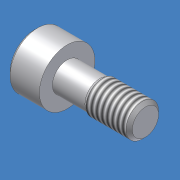
# Autodesk Inventor part: HCBST5-12_Screw
Saved by Autodesk Inventor 2014 SP1 (Build 180222100, 222)
## iProperties
Category: PARTsolutions
Created: 2015-02-04
Part Number: HCBST5-12_Screw
Catalog Web Link: www.cadenas.de
Description: HCBSTscrew - Frame Washer Assembled Hexagon Socket Head Cap Screws for Aluminum Frames
Document SubType Name: Modeling
Designer: PARTsolutions
Material: Generic
Density: 1 g/cm^3
Appearance: RGB(192,192,192)
NB: HCBST5-12_Screw
NN: HCBSTscrew
NT: Frame Washer Assembled Hexagon Socket Head Cap Screws for Aluminum Frames
NBSYN: $PN.
LINA: HCBST5-12_Screw
PN: HCBST5-12_Screw
TYPE: HCBST
MATB: Structural Alloy Steel
HARD: 32~44HRC
MATSW: JIS B1251
MATFW: JIS B1256
ST: Trivalent Chromate
M: 5
L: 12
M1: 5.000
L0: 12,16
NDM: 5.000
KDM: 4.017
MP: 5X0.8
P: 0.800
A: 8.5
E: 5
B: 4
C: 8.5
D: 10.0
AA: 5.4
KT: DUMMY
SUPPLIER: Misumi
ARTICLENO: HCBST5-12_Screw
BOMINFO: HCBST5-12_Screw
CREATOR: CADENAS GmbH
PSOL_IDENT_0: {\\10.0.0.236\data_v8\23d-libs\misumi\metric\38_al_extrusions_blackets\nuts\hcbst_screw.prj},177 {VT
PSOL_IDENT_1: YP=3D},{NB=HCBST5-12_Screw},{LINA=HCBST5-12_Screw},{NN=HCBSTscrew},{DATE=19.11.2014 02:34:01},{GEOMD
PSOL_IDENT_2: ATE=24.08.2009 08:32:00},{VERSION=},{LINEID=40},{LINESUBID=-1},{WBVAR=L}  {NB=HCBST5-12_Screw},{LINA
PSOL_IDENT_3: =HCBST5-12_Screw},{KT=DUMMY},{PN=HCBST5-12_Screw},{TYPE=HCBST},{MATB=Structural Alloy Steel},{HARD=3
PSOL_IDENT_4: 2~44HRC},{MATSW=JIS B1251},{MATFW=JIS B1256},{ST=Trivalent Chromate},{M=5},{L=12},{M1=5.000},{L0=12,
PSOL_IDENT_5: 16},{NDM=5},{KDM=4.017064},{MP=5X0.8},{P=0.8},{A=8.5},{E=5},{B=4},{C=8.5},{D=10.0},{AA=5.4}
Title: HCBST5-12_Screw
Author: Cadenas PARTsolutions
Comments: Frame Washer Assembled Hexagon Socket Head Cap Screws for Aluminum Frames
Autodesk Inventor part; units mm, degrees
sketch "Sketch_6" plane through (0, 0, 0) normal (0, 0, 1) x (1, 0, 0)
  line L0 (12, 0) -> (4.5504, 0)
  line L1 (4.5504, 0) -> (4.5504, 2.0095)
  line L2 (4.5504, 2.0095) -> (5.4, 2.5)
  line L3 (5.4, 2.5) -> (11.5095, 2.5)
  line L4 (11.5095, 2.5) -> (12, 2.0095)
  line L5 (12, 2.0095) -> (12, 0)
  line L6 (12, 0) -> (4.5504, 0)
  constraints: 14 end point
revolve "Revolution1" add sketch "Sketch_6" angle 360 about axis through (12, 0, 0) along (1, 0, 0)
thread "Thread1" size "M5x0.8" class "6g" standard "ISO Metric profile" full length
sketch "Sketch_1" plane through (0, 0, 0) normal (0, 0, 1) x (1, 0, 0)
  line L0 (5.4, 0) -> (-5, 0)
  line L1 (-1.3453, 0) -> (-2.5, 2)
  line L2 (-2.5, 2) -> (-5, 2)
  line L3 (-5, 2) -> (-5, 3.75)
  line L4 (-5, 3.75) -> (-4.5, 4.25)
  line L5 (-4.5, 4.25) -> (0, 4.25)
  line L6 (0, 4.25) -> (0, 2.2543)
  line L7 (0, 2.2543) -> (5.4, 2.2543)
  line L8 (5.4, 2.2543) -> (5.4, 0)
  line L9 (5.4, 0) -> (-1.3453, 0)
  constraints: 20 end point
revolve "Revolution2" add sketch "Sketch_1" angle 360 about axis through (5.4, 0, 0) along (1, 0, 0)
sketch "Sketch_2" plane through (-5, 0, 0) normal (1, 0, 0) x (0, 0, -1)
  line L0 (-2, 1.1547) -> (-2, -1.1547)
  line L1 (-2, -1.1547) -> (0, -2.3094)
  line L2 (0, -2.3094) -> (2, -1.1547)
  line L3 (2, -1.1547) -> (2, 1.1547)
  line L4 (2, 1.1547) -> (0, 2.3094)
  line L5 (0, 2.3094) -> (-2, 1.1547)
  constraints: 12 end point
extrude "Extrusion1" cut sketch "Sketch_2" along normal blind 2.5
ref_plane "bolt_to_spring_washer_XY" through (1.8, 0, 0) normal (1, 0, 0) x (0, 0, -1)
ref_plane "bolt_to_spring_washer_YZ" through (1.8, 0, 0) normal (0, 0, -1) x (0, 1, 0)
ref_plane "bolt_to_spring_washer_ZX" through (1.8, 0, 0) normal (0, 1, 0) x (1, 0, 0)
ref_plane "bolt_to_plane_washer_XY" through (3.6, 0, 0) normal (1, 0, 0) x (0, 0, -1)
ref_plane "bolt_to_plane_washer_YZ" through (3.6, 0, 0) normal (0, 0, -1) x (0, 1, 0)
ref_plane "bolt_to_plane_washer_ZX" through (3.6, 0, 0) normal (0, 1, 0) x (1, 0, 0)
ref_plane "screw_to_body_XY" through (0, 0, 0) normal (1, 0, 0) x (0, 0, -1)
ref_plane "screw_to_body_YZ" through (0, 0, 0) normal (0, 0, -1) x (0, 1, 0)
ref_plane "screw_to_body_ZX" through (0, 0, 0) normal (0, 1, 0) x (1, 0, 0)
body "Solid1"
